Autodesk Fusion 360 part; units mm, degrees
(part 2 of 3)
  spline S18 degree 5 poles (-10, 45) (-11.9791, 46.0284) (-15.9034, 48.1188) (-21.6887, 51.3552) (-29.1964, 55.8754) (-38.2146, 61.8908) (-46.833, 68.3041) (-55.0184, 75.1487) (-62.7516, 82.4437) (-70.0489, 90.1727) (-76.9426, 98.3036) (-82.1609, 105.1037) (-85.9183, 110.3595) (-88.3548, 113.9314) (-89.5561, 115.7344) knots 0 0 0 0 0 0 0.1 0.2 0.3 0.4 0.5 0.6 0.7 0.8 0.9 1 1 1 1 1 1
  arc A19 (-109.3801, 88.0477) -> (-89.5561, 115.7344) centre (-108, 108) ccw
  spline S19 degree 5 poles (-109.3801, 88.0477) (-108.6093, 87.8146) (-105.5101, 86.8635) (-100.1552, 85.1208) (-92.6931, 82.436) (-83.3647, 78.5649) (-73.161, 73.5176) (-63.577, 67.8424) (-54.6474, 61.5042) (-46.356, 54.5193) (-38.6588, 46.9323) (-32.9395, 40.4185) (-28.8813, 35.2989) (-26.2769, 31.7834) (-25, 30) knots -0.932954 -0.932954 -0.932954 -0.932954 -0.932954 -0.932954 -0.9 -0.8 -0.7 -0.6 -0.5 -0.4 -0.3 -0.2 -0.1 0 0 0 0 0 0
  line L518 (-25, 30) -> (-25, -30)
  line L519 (-86.9472, 94.7515) -> (-83.881, 103.9354)
  line L520 (86.9472, 94.7515) -> (83.881, 103.9354)
  line L521 (79.9758, 98.774) -> (86.334, 95.1053)
  line L522 (86.334, 95.1053) -> (86.9472, 94.7515)
  line L523 (-79.314, -96.6555) -> (-78.9776, -97.5027)
  line L524 (-86.9472, -94.7515) -> (-83.881, -103.9354)
  line L525 (-86.334, -95.1053) -> (-86.9472, -94.7515)
  line L526 (-79.9758, -98.774) -> (-86.334, -95.1053)
  line L527 (86.334, -95.1053) -> (86.9472, -94.7515)
  line L528 (78.9776, -97.5027) -> (85.6123, -93.6745)
  line L529 (86.9472, -94.7515) -> (83.881, -103.9354)
  line L530 (79.314, -96.6555) -> (78.9776, -97.5027)
  line L531 (84.24, -103.2596) -> (83.881, -103.9354)
  line L532 (79.9758, -98.774) -> (86.334, -95.1053)
  line L533 (79.1831, -97.3842) -> (85.5398, -93.7163)
  line L534 (86.334, -95.1053) -> (86.9472, -94.7515)
  line L535 (79.9758, -98.774) -> (86.334, -95.1053)
  point P0 (23.3348, -10)
  point P1 (23.3348, 10)
  point P2 (-23.3348, -10)
  point P3 (108, -108)
  point P4 (0, -45)
  point P5 (10, -45)
  point P6 (25, 30)
  point P7 (-108, 108)
  point P8 (10, 45)
  point P9 (0, 45)
  point P10 (0, 45)
  point P11 (-25, 30)
  point P12 (108, 108)
  point P13 (-89.3497, -94.6985)
  point P14 (-77.908, -95.8607)
  point P15 (-90.7737, -97.8385)
  point P16 (-77.8281, -96.0622)
  point P17 (-79.1831, -97.3842)
  point P18 (90.7737, -97.8385)
  point P19 (89.3497, -94.6985)
  point P20 (87.9816, -93.5909)
  point P21 (91.6554, -96.5652)
  point P22 (86.7336, -92.5805)
  point P23 (77.908, -95.8607)
  point P24 (77.8281, -96.0622)
  dimension "d34" = 60
  dimension "d38" = 60
  dimension "d39" = 3
  dimension "d40" = 3
  dimension "d41" = 30.5
  dimension "d49" = 10
  dimension "d50" = 10
  dimension "d52" = 1
  dimension "d82" = 1.6
  dimension "d84" = 1.6
  constraint parallel L0 L1
  constraint parallel L0 L2
  constraint coincident L2 S3.start
  constraint coincident L4 L5.end
  constraint coincident S2 L6.end
  constraint coincident L0 L8.start
  constraint coincident L4 L8.end
  constraint coincident L4 L7.start
  constraint coincident S2 L7.end
  constraint coincident L4 L9.end
  constraint horizontal L10
  constraint coincident L12.start L13.start
  constraint perpendicular L11 L12
  constraint perpendicular L10 L13
  constraint coincident P4 L14
  constraint symmetric L13 A2.centre A3.centre
  constraint symmetric L10.start L11 L15.end
  constraint symmetric L10.end L11 L15.start
  constraint symmetric L13.start L12 L16.start
  constraint symmetric P10 L12 P9
  constraint midpoint L18 L19.start
  constraint midpoint L17 L19.end
  constraint symmetric A2 L19 A4
  constraint symmetric A3 L19 A5
  constraint coincident L19 L20.start
  constraint perpendicular L19 L20
  constraint perpendicular L19 L21
  constraint perpendicular L22 L24
  constraint perpendicular L23 L25
  constraint tangent L22 A6
  constraint tangent L24 A6
  constraint coincident P0 L20
  constraint coincident P0 L24
  constraint tangent L20 A7
  constraint tangent L24 A7
  constraint equal A6 A7
  constraint coincident P1 L21
  constraint coincident P1 L25
  constraint tangent L21 A8
  constraint tangent L25 A8
  constraint equal A6 A8
  constraint tangent L23 A9
  constraint tangent L25 A9
  constraint equal A6 A9
  constraint symmetric L12 L20.start L27.start
  constraint symmetric L12 P0 P2
  constraint symmetric L12 L22.start L26.start
  constraint symmetric L12 L22.end L26.end
  constraint symmetric L12 L24.end L28.end
  constraint symmetric L12 A6 A11
  constraint symmetric L12 L20.end L27.end
  constraint symmetric L12 L24.start A10.end
  constraint symmetric L12 A7 A10
  constraint symmetric L12 L21.end L30.end
  constraint symmetric L12 L25.start A13.start
  constraint symmetric L12 A8 A13
  constraint symmetric L12 L23.end L29.end
  constraint symmetric L12 L25.end A12.end
  constraint symmetric L12 A9 A12
  constraint coincident S2 L33.start
  constraint coincident L4 L34.end
  constraint parallel L33 L34
  constraint coincident S2 L35.end
  constraint vertical L35
  constraint coincident L4 L37.start
  constraint coincident S2 L38.end
  constraint parallel L37 L38
  constraint coincident L4 L39.end
  constraint coincident S2 L40.start
  constraint coincident S3 L40.end
  constraint coincident S2 L42.start
  constraint coincident L4 L43.end
  constraint parallel L42 L43
  constraint coincident S2 L44.end
  constraint coincident L4 L46.start
  constraint coincident S2 L47.end
  constraint parallel L46 L47
  constraint coincident L4 L48.end
  constraint coincident S2 L50.start
  constraint coincident L4 L51.end
  constraint parallel L50 L51
  constraint coincident S2 L52.end
  constraint coincident S3 L53.end
  constraint coincident L4 L54.end
  constraint coincident S2 L55.end
  constraint coincident L4 L56.start
  constraint coincident S2 L57.end
  constraint parallel L56 L57
  constraint coincident L4 L58.end
  constraint coincident S2 L60.start
  constraint coincident L4 L61.end
  constraint parallel L60 L61
  constraint coincident S2 L62.end
  constraint coincident L4 L64.start
  constraint coincident S2 L65.end
  constraint parallel L64 L65
  constraint coincident L4 L66.end
  constraint coincident S2 L68.start
  constraint coincident L4 L69.end
  constraint parallel L68 L69
  constraint coincident S2 L70.end
  constraint coincident L4 L72.start
  constraint coincident S2 L73.end
  constraint parallel L72 L73
  constraint coincident L4 L74.end
  constraint coincident S2 L76.start
  constraint coincident L4 L77.end
  constraint parallel L76 L77
  constraint coincident S2 P16
  constraint coincident L4 L80.start
  constraint coincident S2 L81.end
  constraint parallel L80 L81
  constraint coincident L4 L82.end
  constraint coincident S2 L84.start
  constraint coincident L4 L85.end
  constraint parallel L84 L85
  constraint coincident S2 L87.end
  constraint coincident A0 P15
  constraint coincident A1 P15
  constraint coincident A0 L88.end
  constraint coincident A0 L89.end
  constraint coincident L3 L90.start
  constraint coincident S3 L91.end
  constraint coincident L3 L92.start
  constraint coincident L0 L92.end
  constraint coincident S3 L94.end
  constraint parallel L93 L94
  constraint coincident L3 L93.start
  constraint coincident L3 L95.end
  constraint coincident S3 L96.start
  constraint coincident L3 L97.end
  constraint parallel L96 L97
  constraint coincident S3 L98.end
  constraint coincident L3 L99.start
  constraint coincident S3 L100.end
  constraint parallel L99 L100
  constraint coincident L3 L101.end
  constraint vertical L101
  constraint coincident L3 L103.end
  constraint parallel L102 L103
  constraint coincident S3 L102.start
  constraint coincident S3 L104.end
  constraint coincident L3 L105.start
  constraint coincident S3 L106.end
  constraint parallel L105 L106
  constraint coincident L3 L107.end
  constraint coincident S3 L108.start
  constraint coincident L3 L109.end
  constraint parallel L108 L109
  constraint coincident L3 L111.start
  constraint coincident L53 L111.end
  constraint coincident L53 L112.end
  constraint coincident L4 L112.start
  constraint coincident L3 L113.end
  constraint coincident S3 L114.end
  constraint coincident L3 L115.start
  constraint coincident S3 L116.end
  constraint parallel L115 L116
  constraint coincident L3 L117.end
  constraint parallel L40 L53
  constraint coincident L3 L119.end
  constraint parallel L118 L119
  constraint coincident S3 L120.end
  constraint coincident S3 L118.start
  constraint coincident L3 L121.start
  constraint coincident S3 L122.end
  constraint parallel L121 L122
  constraint coincident L3 L123.end
  constraint coincident L3 L125.end
  constraint parallel L124 L125
  constraint coincident S3 L124.start
  constraint coincident S3 L126.end
  constraint coincident L3 L127.start
  constraint coincident S3 L128.end
  constraint parallel L127 L128
  constraint coincident L3 L129.end
  constraint coincident L3 L131.end
  constraint parallel L130 L131
  constraint coincident S3 L132.end
  constraint parallel L130 L132
  constraint coincident S3 L133.end
  constraint coincident L3 L134.start
  constraint coincident S3 L135.end
  constraint parallel L134 L135
  constraint coincident L3 L136.end
  constraint coincident S3 L138.end
  constraint parallel L137 L138
  constraint coincident S3 L140.end
  constraint coincident A1 L139.end
  constraint coincident L3 L137.end
  constraint coincident L3 P13
  constraint coincident L139 L142.end
  constraint parallel L141 L142
  constraint symmetric S1.end L13 P5
  constraint symmetric S0.end L13 A14.start
  constraint symmetric A0.start L13 A14.end
  constraint symmetric A0 L13 A14
  constraint symmetric S1 L13 S6
  constraint symmetric S3.end L13 S4.end
  constraint symmetric S2.start L13 S5.start
  constraint symmetric L0.end L13 L145.start
  constraint symmetric L0.start L13 L159.start
  constraint symmetric L1.end L13 L159.end
  constraint symmetric L2.end L13 L145.end
  constraint symmetric S2 L13 S5
  constraint symmetric S3 L13 S4
  constraint symmetric A0.centre L13 P3
  constraint symmetric L3.start L13 L201.start
  constraint symmetric L3.end L13 P21
  constraint symmetric L4.start L13 L254.start
  constraint symmetric P15 L13 P18
  constraint symmetric L5.end L13 L168.start
  constraint symmetric L6.end L13 L150.end
  constraint symmetric L8.start L13 L166.start
  constraint symmetric L8.end L13 L166.end
  constraint symmetric L7.start L13 L262.start
  constraint symmetric L7.end L13 L260.start
  constraint symmetric L9.end L13 L260.end
  constraint symmetric P4 L13 L13.end
  constraint symmetric L13 S1.end P5
  constraint symmetric L13 L32.start L150.start
  constraint symmetric L13 L33.end L266.start
  constraint symmetric L13 L33.start L267.start
  constraint symmetric L13 L34.end L160.start
  constraint symmetric L13 L35.end L160.end
  constraint symmetric L13 L36.start L148.start
  constraint symmetric L13 L36.end L147.start
  constraint symmetric L13 L37.end L161.end
  constraint symmetric L13 L37.start L161.start
  constraint symmetric L13 L38.end L245.start
  constraint symmetric L13 L39.end L245.end
  constraint symmetric L13 L40.start L211.start
  constraint symmetric L13 L40.end L212.end
  constraint symmetric L13 L41.start L149.start
  constraint symmetric L13 L41.end L149.end
  constraint symmetric L13 L42.end L162.start
  constraint symmetric L13 L42.start L218.start
  constraint symmetric L13 L43.end L154.start
  constraint symmetric L13 L44.end L154.end
  constraint symmetric L13 L45.start L157.start
  constraint symmetric L13 L45.end L157.end
  constraint symmetric L13 L46.end L165.start
  constraint symmetric L13 L46.start L249.start
  constraint symmetric L13 L47.end L165.end
  constraint symmetric L13 L48.end L199.end
  constraint symmetric L13 L49.start L151.start
  constraint symmetric L13 L49.end L151.end
  constraint symmetric L13 L50.end L155.end
  constraint symmetric L13 L50.start L155.start
  constraint symmetric L13 L51.end L163.end
  constraint symmetric L13 L52.end L198.end
  constraint symmetric L13 L53.end L196.end
  constraint symmetric L13 L54.end L211.end
  constraint symmetric L13 L55.end L250.end
  constraint symmetric L13 L56.end L144.end
  constraint symmetric L13 L56.start L144.start
  constraint symmetric L13 L57.end L190.end
  constraint symmetric L13 L58.end L194.end
  constraint symmetric L13 L59.start L213.start
  constraint symmetric L13 L59.end L213.end
  constraint symmetric L13 L60.end L184.start
  constraint symmetric L13 L60.start L185.start
  constraint symmetric L13 L61.end L184.end
  constraint symmetric L13 L62.end L234.end
  constraint symmetric L13 L63.start L251.start
  constraint symmetric L13 L63.end L183.start
  constraint symmetric L13 L64.end L171.end
  constraint symmetric L13 L64.start L171.start
  constraint symmetric L13 L65.end L233.start
  constraint symmetric L13 L66.end L233.end
  constraint symmetric L13 L67.start L179.start
  constraint symmetric L13 L67.end L179.end
  constraint symmetric L13 L68.end L172.end
  constraint symmetric L13 L68.start L172.start
  constraint symmetric L13 L69.end L236.end
  constraint symmetric L13 L70.end L240.end
  constraint symmetric L13 L71.start L176.start
  constraint symmetric L13 L71.end L176.end
  constraint symmetric L13 L72.end L175.start
  constraint symmetric L13 L72.start L180.start
  constraint symmetric L13 L73.end L174.start
  constraint symmetric L13 L74.end L174.end
  constraint symmetric L13 L75.start L238.start
  constraint symmetric L13 L75.end L238.end
  constraint symmetric L13 L76.end L170.start
  constraint symmetric L13 L76.start L177.start
  constraint symmetric L13 L77.end L169.start
  constraint symmetric L13 P16 P24
  constraint symmetric L13 L79.start L173.start
  constraint symmetric L13 L79.end L173.end
  constraint symmetric L13 L80.end L186.end
  constraint symmetric L13 L80.start L186.start
  constraint symmetric L13 L81.end L241.end
  constraint symmetric L13 L82.end L244.end
  constraint symmetric L13 L83.start L237.start
  constraint symmetric L13 P14 P23
  constraint symmetric L13 L84.end L143.end
  constraint symmetric L13 L84.start L143.start
  constraint symmetric L13 L85.end L231.end
  constraint symmetric L13 P17 L191.start
  constraint symmetric L13 L86.end L191.end
  constraint symmetric L13 L87.start L225.start
  constraint symmetric L13 L87.end L222.start
  constraint symmetric L13 L88.end L228.end
  constraint symmetric L13 L89.start L206.start
  constraint symmetric L13 L89.end L206.end
  constraint symmetric L13 L90.start L146.start
  constraint symmetric L13 L91.end L146.end
  constraint symmetric L13 L92.start L264.start
  constraint symmetric L13 L92.end L264.end
  constraint symmetric L13 L93.end L256.start
  constraint symmetric L13 L94.end L255.start
  constraint symmetric L13 L93.start L263.start
  constraint symmetric L13 L95.end L147.end
  constraint symmetric L13 L96.end L248.end
  constraint symmetric L13 L96.start L248.start
  constraint symmetric L13 L97.end L246.start
  constraint symmetric L13 L98.end L246.end
  constraint symmetric L13 L99.end L153.start
  constraint symmetric L13 L99.start L247.start
  constraint symmetric L13 L100.end L153.end
  constraint symmetric L13 L101.end L158.end
  constraint symmetric L13 L102.end L215.start
  constraint symmetric L13 L103.end L215.end
  constraint symmetric L13 L102.start L219.start
  constraint symmetric L13 L104.end L217.end
  constraint symmetric L13 L105.end L167.start
  constraint symmetric L13 L105.start L220.start
  constraint symmetric L13 L106.end L156.start
  constraint symmetric L13 L107.end L156.end
  constraint symmetric L13 L108.end L152.start
  constraint symmetric L13 L108.start L197.start
  constraint symmetric L13 L109.end L152.end
  constraint symmetric L13 L111.start L216.start
  constraint symmetric L13 L111.end L216.end
  constraint symmetric L13 L112.end L195.end
  constraint symmetric L13 L112.start L195.start
  constraint symmetric L13 L113.end L188.start
  constraint symmetric L13 L114.end L188.end
  constraint symmetric L13 L115.end L189.start
  constraint symmetric L13 L115.start L209.start
  constraint symmetric L13 L116.end L181.start
  constraint symmetric L13 L117.end L181.end
  constraint symmetric L13 L118.end L182.end
  constraint symmetric L13 L119.end L210.start
  constraint symmetric L13 L120.end L210.end
  constraint symmetric L13 L118.start L182.start
  constraint symmetric L13 L121.end L193.start
  constraint symmetric L13 L121.start L214.start
  constraint symmetric L13 L122.end L193.end
  constraint symmetric L13 L123.end L242.end
  constraint symmetric L13 L124.end L178.start
  constraint symmetric L13 L125.end L178.end
  constraint symmetric L13 L124.start L239.start
  constraint symmetric L13 L126.end L187.end
  constraint symmetric L13 L127.end L205.start
  constraint symmetric L13 L127.start L243.start
  constraint symmetric L13 L128.end L192.start
  constraint symmetric L13 L129.end L192.end
  constraint symmetric L13 L130.start L203.start
  constraint symmetric L13 L130.end L224.end
  constraint symmetric L13 L131.end L204.start
  constraint symmetric L13 L132.end L203.end
  constraint symmetric L13 L133.end L204.end
  constraint symmetric L13 L134.end L208.start
  constraint symmetric L13 L134.start L232.start
  constraint symmetric L13 L135.end L207.start
  constraint symmetric L13 L136.end P22
  constraint symmetric L13 L137.start L227.start
  constraint symmetric L13 L137.end P20
  constraint symmetric L13 L138.end L227.end
  constraint symmetric L13 L140.end L221.end
  constraint symmetric L13 L139.end L223.end
  constraint symmetric L13 L141.end L202.end
  constraint symmetric L13 P13 P19
  constraint symmetric L13 L142.end L226.end
  constraint symmetric S1.end L19 L272.end
  constraint symmetric S0.start L19 P11
  constraint symmetric S0.end L19 S8.end
  constraint symmetric S0 L19 S8
  constraint symmetric A0.start L19 S7.start
  constraint symmetric A0 L19 A15
  constraint symmetric S1 L19 S7
  constraint symmetric S3.end L19 L431.start
  constraint symmetric S2.start L19 L385.start
  constraint symmetric L0.end L19 L364.start
  constraint symmetric L0.start L19 L435.start
  constraint symmetric L1.end L19 L339.start
  constraint symmetric L2.end L19 L364.end
  constraint symmetric S2 L19 S12
  constraint symmetric S3 L19 S13
  constraint symmetric A0.centre L19 P7
  constraint symmetric L3.start L19 L464.start
  constraint symmetric L3.end L19 L464.end
  constraint symmetric L4.start L19 L341.start
  constraint symmetric P15 L19 L341.end
  constraint symmetric L5.end L19 L339.end
  constraint symmetric L6.end L19 L382.end
  constraint symmetric L8.start L19 L444.start
  constraint symmetric L8.end L19 L444.end
  constraint symmetric L7.start L19 L419.start
  constraint symmetric L7.end L19 L419.end
  constraint symmetric L9.end L19 L443.end
  constraint symmetric P4 L19 P10
  constraint symmetric P5 L19 P8
  constraint symmetric L18.end L19 P6
  constraint symmetric L19 L32.start L421.start
  constraint symmetric L19 L33.end L413.start
  constraint symmetric L19 L33.start L437.start
  constraint symmetric L19 L34.end L413.end
  constraint symmetric L19 L35.end L457.end
  constraint symmetric L19 L36.start L404.start
  constraint symmetric L19 L36.end L373.start
  constraint symmetric L19 L37.end L438.start
  constraint symmetric L19 L37.start L461.start
  constraint symmetric L19 L38.end L438.end
  constraint symmetric L19 L39.end L468.end
  constraint symmetric L19 L40.start L345.start
  constraint symmetric L19 L40.end L345.end
  constraint symmetric L19 L41.start L352.start
  constraint symmetric L19 L41.end L352.end
  constraint symmetric L19 L42.end L360.start
  constraint symmetric L19 L42.start L410.start
  constraint symmetric L19 L43.end L360.end
  constraint symmetric L19 L44.end L416.end
  constraint symmetric L19 L45.start L391.start
  constraint symmetric L19 L45.end L391.end
  constraint symmetric L19 L46.end L362.end
  constraint symmetric L19 L46.start L362.start
  constraint symmetric L19 L47.end L369.start
  constraint symmetric L19 L48.end L369.end
  constraint symmetric L19 L49.start L397.start
  constraint symmetric L19 L49.end L397.end
  constraint symmetric L19 L50.end L407.end
  constraint symmetric L19 L50.start L407.start
  constraint symmetric L19 L51.end L423.end
  constraint symmetric L19 L52.end L436.end
  constraint symmetric L19 L53.end L342.end
  constraint symmetric L19 L54.end L354.end
  constraint symmetric L19 L55.end L361.end
  constraint symmetric L19 L56.end L383.end
  constraint symmetric L19 L56.start L383.start
  constraint symmetric L19 L57.end L344.start
  constraint symmetric L19 L58.end L344.end
  constraint symmetric L19 L59.start L376.start
  constraint symmetric L19 L59.end L376.end
  constraint symmetric L19 L60.end L363.start
  constraint symmetric L19 L60.start L370.start
  constraint symmetric L19 L61.end L346.start
  constraint symmetric L19 L62.end L346.end
  constraint symmetric L19 L63.start L470.start
  constraint symmetric L19 L63.end L350.start
  constraint symmetric L19 L64.end L377.start
  constraint symmetric L19 L64.start L399.start
  constraint symmetric L19 L65.end L375.start
  constraint symmetric L19 L66.end L375.end
  constraint symmetric L19 L67.start L411.start
  constraint symmetric L19 L67.end L411.end
  constraint symmetric L19 L68.end L392.start
  constraint symmetric L19 L68.start L396.start
  constraint symmetric L19 L69.end L392.end
  constraint symmetric L19 L70.end L424.end
  constraint symmetric L19 L71.start L420.start
  constraint symmetric L19 L71.end L420.end
  constraint symmetric L19 L72.end L395.start
  constraint symmetric L19 L72.start L406.start
  constraint symmetric L19 L73.end L359.start
  constraint symmetric L19 L74.end L359.end
  constraint symmetric L19 L75.start L401.start
  constraint symmetric L19 L75.end L401.end
  constraint symmetric L19 L76.end L394.start
  constraint symmetric L19 L76.start L414.start
  constraint symmetric L19 L77.end L394.end
  constraint symmetric L19 P16 L409.end
  constraint symmetric L19 L79.start L384.start
  constraint symmetric L19 L79.end L384.end
  constraint symmetric L19 L80.end L368.end
  constraint symmetric L19 L80.start L368.start
  constraint symmetric L19 L81.end L405.end
  constraint symmetric L19 L82.end L472.end
  constraint symmetric L19 L83.start L403.start
  constraint symmetric L19 P14 L403.end
  constraint symmetric L19 L84.end L428.start
  constraint symmetric L19 L84.start L471.start
  constraint symmetric L19 L85.end L428.end
  constraint symmetric L19 P17 L465.start
  constraint symmetric L19 L86.end L465.end
  constraint symmetric L19 L87.end L519.end
  constraint symmetric L19 L88.end L385.end
  constraint symmetric L19 L90.start L456.end
  constraint symmetric L19 L91.end L460.end
  constraint symmetric L19 L92.start L459.start
  constraint symmetric L19 L92.end L459.end
  constraint symmetric L19 L93.end L365.start
  constraint symmetric L19 L94.end L365.end
  constraint symmetric L19 L93.start L426.start
  constraint symmetric L19 L95.end L373.end
  constraint symmetric L19 L96.end L434.start
  constraint symmetric L19 L96.start L469.start
  constraint symmetric L19 L97.end L434.end
  constraint symmetric L19 L98.end L466.end
  constraint symmetric L19 L99.end L353.end
  constraint symmetric L19 L99.start L353.start
  constraint symmetric L19 L100.end L349.start
  constraint symmetric L19 L101.end L349.end
  constraint symmetric L19 L102.end L412.end
  constraint symmetric L19 L103.end L415.start
  constraint symmetric L19 L102.start L412.start
  constraint symmetric L19 L104.end L415.end
  constraint symmetric L19 L105.end L380.start
  constraint symmetric L19 L105.start L439.start
  constraint symmetric L19 L106.end L380.end
  constraint symmetric L19 L107.end L433.end
  constraint symmetric L19 L108.end L351.start
  constraint symmetric L19 L108.start L389.start
  constraint symmetric L19 L109.end L342.start
  constraint symmetric L19 L111.start L393.start
  constraint symmetric L19 L111.end L393.end
  constraint symmetric L19 L112.end L398.end
  constraint symmetric L19 L112.start L398.start
  constraint symmetric L19 L113.end L355.end
  constraint symmetric L19 L114.end L402.end
  constraint symmetric L19 L115.end L347.start
  constraint symmetric L19 L115.start L379.start
  constraint symmetric L19 L116.end L347.end
  constraint symmetric L19 L117.end L350.end
  constraint symmetric L19 L118.end L356.end
  constraint symmetric L19 L119.end L371.start
  constraint symmetric L19 L120.end L371.end
  constraint symmetric L19 L118.start L356.start
  constraint symmetric L19 L121.end L358.end
  constraint symmetric L19 L121.start L358.start
  constraint symmetric L19 L122.end L343.start
  constraint symmetric L19 L123.end L343.end
  constraint symmetric L19 L124.end L366.end
  constraint symmetric L19 L125.end L367.start
  constraint symmetric L19 L124.start L366.start
  constraint symmetric L19 L126.end L367.end
  constraint symmetric L19 L127.end L357.end
  constraint symmetric L19 L127.start L357.start
  constraint symmetric L19 L128.end L430.end
  constraint symmetric L19 L129.end L467.end
  constraint symmetric L19 L130.start L400.start
  constraint symmetric L19 L130.end L400.end
  constraint symmetric L19 L131.end L417.start
  constraint symmetric L19 L132.end L422.end
  constraint symmetric L19 L133.end L417.end
  constraint symmetric L19 L134.end L390.start
  constraint symmetric L19 L134.start L441.start
  constraint symmetric L19 L135.end L390.end
  constraint symmetric L19 L136.end L432.end
  constraint symmetric L19 L137.start L381.start
  constraint symmetric L19 L137.end L381.end
  constraint symmetric L19 L138.end L425.end
  constraint symmetric L19 L140.end L408.end
  constraint symmetric L19 L139.end L431.end
  constraint symmetric L19 L141.end L348.start
  constraint symmetric L19 P13 L387.start
  constraint symmetric L19 L142.end L348.end
  constraint symmetric L19 L231.end L488.end
  constraint symmetric L19 L143.start L455.start
  constraint symmetric L19 L222.start L493.end
  constraint symmetric L19 L176.start L310.start
  constraint symmetric L19 P3 P12
  constraint symmetric L19 L165.end L275.end
  constraint symmetric L19 L176.end L310.end
  constraint symmetric L19 L199.end L290.end
  constraint symmetric L19 L179.start L500.start
  constraint symmetric L19 S5.start S10.start
  constraint symmetric L19 L213.start L508.start
  constraint symmetric L19 P4 P10
  constraint symmetric L19 L249.start L287.start
  constraint symmetric L19 L165.start L275.start
  constraint symmetric L19 L196.end L300.end
  constraint symmetric L19 L215.start L289.end
  constraint symmetric L19 L228.end L494.end
  constraint symmetric L19 L188.start L496.start
  constraint symmetric L19 L195.start L332.start
  constraint symmetric L19 L195.end L332.end
  constraint symmetric L19 L188.end L496.end
  constraint symmetric L19 L216.start L291.start
  constraint symmetric L19 L216.end L291.end
  constraint symmetric L19 L172.start L316.start
  constraint symmetric L19 L225.start L493.start
  constraint symmetric L19 L209.start L507.start
  constraint symmetric L19 L182.end L504.start
  constraint symmetric L19 L181.start L509.end
  constraint symmetric L19 L210.start L303.start
  constraint symmetric L19 L182.start L510.start
  constraint symmetric L19 L189.start L507.end
  constraint symmetric L19 L181.end L511.end
  constraint symmetric L19 L214.start L315.start
  constraint symmetric L19 L244.end L454.end
  constraint symmetric L19 P20 L446.start
  constraint symmetric L19 P22 L487.end
  constraint symmetric L19 L143.end L455.end
  constraint symmetric L19 L203.start L447.start
  constraint symmetric L19 L233.start L304.start
  constraint symmetric L19 L242.end L474.end
  constraint symmetric L19 L193.end L313.end
  constraint symmetric L19 L203.end L490.end
  constraint symmetric L19 L204.end L453.end
  constraint symmetric L19 L246.start L280.start
  constraint symmetric L19 L246.end L280.end
  constraint symmetric L19 L153.start L320.end
  constraint symmetric L19 L221.end L446.end
  constraint symmetric L19 L208.start L317.start
  constraint symmetric L19 L193.start L313.start
  constraint symmetric L19 L227.end L489.end
  constraint symmetric L19 L248.end L281.start
  constraint symmetric L19 L202.end L491.start
  constraint symmetric L19 A14.end S11.start
  constraint symmetric L19 L178.start L309.start
  constraint symmetric L19 L186.end L311.start
  constraint symmetric L19 A14.start A16.end
  constraint symmetric L19 L248.start L301.start
  constraint symmetric L19 L204.start L306.end
  constraint symmetric L19 L177.start L477.start
  constraint symmetric L19 L224.end L306.start
  constraint symmetric L19 P24 L478.end
  constraint symmetric L19 L227.start L450.start
  constraint symmetric L19 P19 L492.start
  constraint symmetric L19 L207.start L317.end
  constraint symmetric L19 L178.end L309.end
  constraint symmetric L19 L241.end L311.end
  constraint symmetric L19 L239.start L482.start
  constraint symmetric L19 L149.start L331.start
  constraint symmetric L19 L150.start L330.start
  constraint symmetric L19 L145.end L268.end
  constraint symmetric L19 L160.start L285.end
  constraint symmetric L19 L201.start L338.start
  constraint symmetric L19 L160.end L299.end
  constraint symmetric L19 S4.end L449.start
  constraint symmetric L19 L254.start L340.start
  constraint symmetric L19 L147.start L270.end
  constraint symmetric L19 L263.start L286.start
  constraint symmetric L19 L151.start L319.start
  constraint symmetric L19 L157.end L321.end
  constraint symmetric L19 L266.start L276.end
  constraint symmetric L19 L158.end L279.end
  constraint symmetric L19 L148.start L270.start
  constraint symmetric L19 L151.end L319.end
  constraint symmetric L19 L159.end L269.end
  constraint symmetric L19 L152.end L297.end
  constraint symmetric L19 P5 P8
  constraint symmetric L19 L260.end L327.end
  constraint symmetric L19 L171.end L479.end
  constraint symmetric L19 L223.end L449.end
  constraint symmetric L19 L185.start L497.start
  constraint symmetric L19 L184.end L473.start
  constraint symmetric L19 L234.end L473.end
  constraint symmetric L19 L171.start L479.start
  constraint symmetric L19 L183.start L502.end
  constraint symmetric L19 L161.start L296.start
  constraint symmetric L19 L218.start L322.start
  constraint symmetric L19 L154.start L278.start
  constraint symmetric L19 L153.end L279.start
  constraint symmetric L19 L267.start L276.start
  constraint symmetric L19 L175.start L307.end
  constraint symmetric L19 L262.start L329.start
  constraint symmetric L19 L180.start L307.start
  constraint symmetric L19 L161.end L296.end
  constraint symmetric L19 L233.end L304.end
  constraint symmetric L19 L162.start L302.start
  constraint symmetric L19 L264.end L273.end
  constraint symmetric L19 L260.start L327.start
  constraint symmetric L19 L245.end L284.end
  constraint symmetric L19 L174.start L481.end
  constraint symmetric L19 L236.end L305.start
  constraint symmetric L19 L172.end L316.end
  constraint symmetric L19 L264.start L273.start
  constraint symmetric L19 L146.start L268.start
  constraint symmetric L19 L245.start L284.start
  constraint symmetric L19 L240.end L305.end
  constraint symmetric L19 L166.end L274.end
  constraint symmetric L19 L154.end L278.end
  constraint symmetric L19 L166.start L274.start
  constraint symmetric L19 L174.end L485.end
  constraint symmetric L19 L150.end L325.end
  constraint symmetric L19 L146.end L277.end
  constraint symmetric L19 L159.start L269.start
  constraint symmetric L19 L145.start L326.end
  constraint symmetric L19 L256.start L282.start
  constraint symmetric L19 L186.start L475.start
  constraint symmetric L19 L232.start L445.start
  constraint symmetric L19 L226.end L491.end
  constraint symmetric L19 L168.start L271.start
  constraint symmetric L19 L169.start L314.end
  constraint symmetric L19 L147.end L283.end
  constraint symmetric L19 L247.start L320.start
  constraint symmetric L19 L210.end L303.end
  constraint symmetric L19 L255.start L282.end
  constraint symmetric L19 L170.start L314.start
  constraint symmetric L19 L173.end L480.end
  constraint symmetric L19 L157.start L321.start
  constraint symmetric L19 L152.start L297.start
  constraint symmetric L19 L197.start L335.start
  constraint symmetric L19 L156.end L295.end
  constraint symmetric L19 L149.end L331.end
  constraint symmetric L19 L238.start L483.start
  constraint symmetric L19 L219.start L289.start
  constraint symmetric L19 L238.end L483.end
  constraint symmetric L19 L156.start L293.end
  constraint symmetric L19 L217.end L336.end
  constraint symmetric L19 L215.end L294.end
  constraint symmetric L19 L220.start L323.start
  constraint symmetric L19 L237.start L476.start
  constraint symmetric L19 L167.start L293.start
  constraint symmetric L19 L251.start L502.start
  constraint symmetric L19 L187.end L312.end
  constraint symmetric L19 L205.start L308.end
  constraint symmetric L19 L243.start L308.start
  constraint symmetric L19 L192.end L451.end
  constraint symmetric L19 L192.start L448.end
  constraint symmetric L19 L191.start L452.start
  constraint symmetric L19 P23 L476.end
  constraint symmetric L19 L211.end L499.start
  constraint symmetric L19 L173.start L480.start
  constraint symmetric L19 L163.end L288.start
  constraint symmetric L19 L155.end L324.end
  constraint symmetric L19 L212.end L498.end
  constraint symmetric L19 P21 L338.end
  constraint symmetric L19 L250.end L499.end
  constraint symmetric L19 L179.end L500.end
  constraint symmetric L19 L198.end L288.end
  constraint symmetric L19 L213.end L508.end
  constraint symmetric L19 L211.start L498.start
  constraint symmetric L19 L190.end L495.end
  constraint symmetric L19 P18 L340.end
  constraint symmetric L19 L144.start L501.start
  constraint symmetric L19 L194.end L512.end
  constraint symmetric L19 L191.end L452.end
  constraint symmetric L19 L184.start L497.end
  constraint symmetric L19 L155.start L324.start
  constraint symmetric L19 L144.end L495.start
  constraint symmetric L19 S4 S9
  constraint symmetric L19 S5 S10
  constraint symmetric L19 A14 A16
  constraint symmetric L19 S6 S11
  constraint symmetric L12 L428.start L455.end
  constraint symmetric L12 L471.start L455.start
  constraint symmetric L12 L428.end L488.end
  constraint symmetric L12 L519.end L493.end
  constraint symmetric L19 L455.end L143.end
  constraint symmetric L19 L493.start L225.start
  constraint symmetric L19 L493.end L222.start
  constraint symmetric L19 L488.end L231.end
  constraint symmetric L19 L340.end P18
  constraint symmetric L19 L446.start P20
  constraint symmetric L19 L311.end L241.end
  constraint symmetric L19 L311.start L186.end
  constraint symmetric L19 L478.end P24
  constraint symmetric L19 L476.end P23
  constraint symmetric L19 L452.start L191.start
  constraint symmetric L19 L465.start P17
  constraint symmetric L19 L341.end P15
  constraint symmetric L19 L403.end P14
  constraint symmetric L19 L387.start P13
  constraint symmetric L19 L368.end L80.end
  constraint symmetric L19 L409.end P16
  constraint symmetric L19 L405.end L81.end
  constraint symmetric L19 L428.start L84.end
  constraint symmetric L19 L471.start L84.start
  constraint symmetric L19 L428.end L85.end
  constraint symmetric L19 L519.end L87.end
  constraint symmetric L19 L338.end P21
  constraint symmetric L19 L455.start L143.start
  constraint symmetric L19 L452.end L191.end
  constraint symmetric L19 L492.start P19
  constraint symmetric L19 L487.end P22
  constraint symmetric L19 L454.end L244.end
  measures "d34" angle of L5 L6
  measures "d38" angle of L4 L7
  measures "d39" diameter of A2
  measures "d40" diameter of A3
  measures "d41" horizontal distance of A2.centre A3.centre
  measures "d49" distance of L20.start P0
  measures "d50" distance of L20.start P1
  measures "d52" radius of A6
  measures "d150" diameter of L9.end
extrude "Extrude3" cut sketch "Sketch5" against normal blind 15 contours S2 L50 L51 L52 | S3 L108 L109 L110 | L4 L46 L47 L48 | L3 L105 L106 L107 | S2 L42 L43 L44 L49 | S3 L102 L103 L104 | L4 L37 L38 L39 L45 | L3 L99 L100 L101 | S2 L33 L34 L35 L41 | S3 L96 L97 L98 | L4 L7 L9 L36 | L3 L93 L94 L95 | S2 L5 L6 L32 | S3 L90 L91 bodies 1
sketch "Sketch7" plane through (0, 0, 6) normal (0, 0, 1) x (-1, 0, 0)
  circle A0 centre (108, 108) radius 20
  circle A1 centre (-108, 108) radius 20
  circle A2 centre (-108, -108) radius 20
  circle A3 centre (108, -108) radius 20
extrude "Extrude4" cut sketch "Sketch5" against normal blind 15 contours S2 L84 L85 L524 L525 L526 | S3 L137 L138 L140 | L4 L80 L81 L82 L86 L523 | L3 L134 L135 L136 | S2 L76 L77 L78 L83 | S3 L130 L131 L132 L133 | L4 L72 L73 L74 L79 | L3 L127 L128 L129 | S2 L68 L69 L70 L75 | S3 L124 L125 L126 | L4 L64 L65 L66 L71 | L3 L121 L122 L123 | S2 L60 L61 L62 L67 | S3 L118 L119 L120 | L4 L56 L57 L58 L63 | L3 L115 L116 L117 | S2 L54 L55 L59 | S3 L113 L114 bodies 1
extrude "Extrude5" cut sketch "Sketch5" against normal blind 15 contours L143 S5 L231 L527 L529 L532 L534 L535 | L186 L191 L241 L244 L254 L528 L530 L533 | S4 L221 L227 L229 | L169 L170 L177 S5 L237 | L201 L207 L208 L232 | L173 L174 L175 L180 L254 | L203 L204 S4 L224 L230 | L172 S5 L236 L238 L240 | L192 L201 L205 L243 | L171 L176 L233 L235 L254 | L178 L187 S4 L239 | L179 L184 L185 S5 L234 | L193 L201 L214 L242 | L144 L190 L194 L251 L254 | L182 S4 L210 L253 | S5 L211 L213 L250 | L181 L189 L201 L209 | L188 S4 L252 bodies 1
extrude "Extrude6" cut sketch "Sketch5" against normal blind 15 contours L155 L163 L198 S5 | L165 L199 L249 L254 | L152 L196 L197 S4 | L151 L154 L162 S5 L218 | L156 L167 L201 L220 | L157 L161 L245 L254 L258 | S4 L215 L217 L219 | L149 L160 S5 L266 L267 | L153 L158 L201 L247 | L148 L254 L260 L262 | S4 L246 L248 L257 | L150 S5 L259 L261 | L201 L255 L256 L263 | L146 S4 L265 bodies 1
extrude "Extrude7" add sketch "Sketch1" along normal blind 6 contours A3 L24 | A3 L24 L26 | A2 L20 L22 | A2 L22 | A3 S7 L26 | A2 S4 L20 | A0 S1 L16 | A1 S3 L18 | A0 L12 L16 | A0 L12 | A1 L14 | A1 L14 L18 bodies 1
sketch "Sketch8" plane through (0, 0, 6) normal (0, 0, 1) x (-1, 0, 0)
  circle A0 centre (108, -108) radius 17
  dimension "d96" = 34
  measures "d96" diameter of A0
extrude "Extrude9" cut sketch "Sketch5" against normal blind 19 contours L19 L29 A12 L30 A13 L31 | L19 L26 L27 A10 L28 A11 | L19 L21 L23 L25 A8 A9 | L19 L20 L22 L24 A6 A7 bodies 1
ref_plane "WorkPlane1" through (0, 0, -30) normal (0, 0, 1) x (1, 0, 0)
sketch "Sketch9" plane through (0, 0, -30) normal (0, 0, 1) x (1, 0, 0)
  line L0 (25, 50) -> (-25, 50)
  line L1 (-25, 50) -> (-25, -50)
  line L2 (-25, -50) -> (25, -50)
  line L3 (25, -50) -> (25, 50)
  line L4 (25, 50) -> (-25, -50) construction
  line L5 (-25, 50) -> (25, -50) construction
  dimension "d102" = 50
  dimension "d103" = 100
  constraint horizontal L0
  constraint perpendicular L0 L1
  constraint parallel L0 L2
  constraint parallel L1 L3
  constraint coincident L4 origin
  constraint coincident L5 origin
  measures "d102" distance of L1.end L2.end
  measures "d103" distance of L0.end L1.end
extrude "Extrude12" add sketch "Sketch9" along normal blind 2.5 separate body makes body 2
sketch "Sketch11" plane through (0, 0, -27.5) normal (0, 0, 1) x (-1, 0, 0)
  line L0 (-25, 50) -> (-25, -50)
  line L1 (-25, -50) -> (25, -50)
  line L2 (25, -50) -> (25, 50)
  line L3 (25, 50) -> (-25, 50)
  circle A0 centre (17, -34) radius 2.5
  line L4 (0, -2.5) -> (0, -20)
  circle A1 centre (-17, -34) radius 2.5
  line L5 (-20, 0) -> (-2.5, 0)
  circle A2 centre (17, 34) radius 2.5
  circle A3 centre (-17, 34) radius 2.5
  dimension "d111" = 5
  constraint symmetric A0 L4 A1
  constraint symmetric A0 L5 A2
  constraint symmetric A1 L5 A3
  measures "d111" diameter of A0
extrude "Extrude13" add sketch "Sketch11" along normal blind 27.5 contours A0 | A1 | A2 | A3 bodies 1 2
extrude "Extrude14" cut sketch "Sketch5" against normal blind 33 contours L455 S10 L488 L520 L521 L522 | L311 L340 L452 L454 L475 | L446 L450 S9 L489 | L314 S10 L476 L477 L478 | L317 L338 L445 L487 | L307 L340 L480 L481 L485 | L306 L447 L453 S9 L490 | L305 L316 S10 L483 L486 | L308 L338 L448 L451 | L304 L310 L340 L479 L484 | L309 L312 S9 L482 | S10 L473 L497 L500 L503 | L313 L315 L338 L474 | L340 L495 L501 L502 L512 | L303 S9 L504 L510 | S10 L499 L506 L508 | L338 L507 L509 L511 | L288 L324 L333 S10 | S9 L496 L514 | L275 L287 L290 L340 | L297 L318 L335 S9 | L278 L302 L319 L322 S10 | L293 L295 L323 L338 | L284 L296 L298 L321 L340 | L289 L294 L336 S9 | L276 L285 L299 L331 S10 | L279 L320 L334 L338 | L270 L327 L329 L340 | L280 L281 L301 S9 | L325 L330 L337 S10 | L282 L286 L292 L338 | L268 L277 S9 bodies 1
extrude "Extrude15" cut sketch "Sketch5" against normal blind 10 contours L381 L408 L425 S13 | L341 L368 L405 L465 L472 | L390 L432 L441 L464 | L394 L403 L409 L414 S12 | L400 L417 L422 L429 S13 | L341 L359 L384 L395 L406 | L357 L430 L464 L467 | L392 L396 L401 L424 S12 | L366 L367 L427 S13 | L341 L375 L377 L399 L420 | L343 L358 L372 L464 | L346 L363 L370 L411 S12 | L356 L371 L374 S13 | L341 L344 L383 L386 L470 | L347 L378 L379 L464 | L354 L361 L376 S12 | L355 L402 S13 | L407 L423 L436 S12 | L342 L351 L389 S13 | L341 L362 L369 L440 | L380 L433 L439 L464 | L360 L397 L410 L416 S12 | L412 L415 L418 S13 | L341 L391 L438 L461 L468 | L349 L353 L388 L464 | L352 L413 L437 L457 S12 | L434 L466 L469 S13 | L341 L404 L419 L443 | L365 L426 L463 L464 | L339 L382 L421 S12 | L458 L460 S13 bodies 1